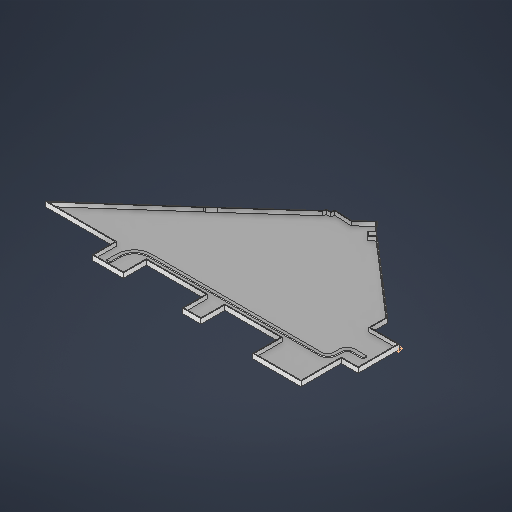
# Autodesk Inventor part: CIT-Floor-2
Saved by Autodesk Inventor 2026.1 (Build 301233020, 233B)
## iProperties
Created: 2025-10-17
Part Number: CIT-Floor-2
Material: Generic
Document SubType Name: Modeling
Designer: eduar
Density: 1 g/cm^3
Appearance: Default
Author: eduar
Autodesk Inventor part; units mm, degrees
ref_plane "YZ Plane" through (0, 0, 0) normal (1, 0, 0) x (0, 1, 0)
ref_plane "XZ Plane" through (0, 0, 0) normal (0, 1, 0) x (-1, 0, 0)
ref_plane "XY Plane" through (0, 0, 0) normal (0, 0, 1) x (1, 0, 0)
sketch "Sketch3" plane through (0, 0, 0) normal (0, 1, 0) x (-1, 0, 0)
  line L0 (0, 10031.5014) -> (4309.3277, 10031.5014)
  line L1 (4309.3277, 10031.5014) -> (4309.3277, 20253.6648)
  line L2 (16182.1297, 20253.6648) -> (4309.3277, 20253.6648)
  line L3 (16182.1297, 13144.1594) -> (16182.1297, 20253.6648)
  line L4 (0, 10031.5014) -> (0, 0)
  line L5 (0, 0) -> (7328.3017, 0)
  line L6 (7328.3017, -4479.3991) -> (7328.3017, 0)
  line L7 (7328.3017, -4479.3991) -> (26439.8438, -20982.2659)
  line L8 (26439.8438, -20982.2659) -> (27514.1147, -19948.948)
  line L9 (27514.1147, -19948.948) -> (28683.7243, -21071.6922)
  line L10 (27775.3508, -22022.2319) -> (28683.7243, -21071.6922)
  line L11 (27775.3508, -22022.2319) -> (29693.6379, -24167.9805)
  line L12 (29693.6379, -24167.9805) -> (32967.4576, -21145.3793)
  line L13 (32967.4576, -21145.3793) -> (37377.4906, -21381.4102)
  line L14 (37377.4906, -21381.4102) -> (37524.0883, -20493.0402)
  line L15 (38604.8798, -20527.5304) -> (37524.0883, -20493.0402)
  line L16 (38604.8798, -20527.5304) -> (38871.047, -19708.2796)
  line L17 (38871.047, -19708.2796) -> (39143.6329, -19289.1159)
  line L18 (39143.6329, -19289.1159) -> (52592.2756, -7382.5123)
  line L19 (38871.047, -19708.2796) -> (52965.6227, -7049.9272)
  line L20 (52965.6227, -7049.9272) -> (54462.7042, -5723.7531)
  line L21 (54850.5695, -5375.3135) -> (54462.7042, -5723.7531)
  line L22 (75709.6936, 13144.1594) -> (54850.5695, -5375.3135)
  line L23 (75709.6936, 13144.1594) -> (58320.151, 13144.1594)
  line L24 (58320.151, 13144.1594) -> (58320.151, 18979.1233)
  line L25 (50758.8526, 18979.1233) -> (58320.151, 18979.1233)
  line L26 (50758.8526, 13144.1594) -> (50758.8526, 18979.1233)
  line L27 (50758.8526, 13144.1594) -> (35157.7821, 13144.1594)
  line L28 (35157.7821, 19212.683) -> (35157.7821, 13144.1594)
  line L29 (30800.956, 19212.683) -> (35157.7821, 19212.683)
  line L30 (30800.956, 13144.1594) -> (30800.956, 19212.683)
  line L31 (30800.956, 13144.1594) -> (16182.1297, 13144.1594)
  dimension "d0" = 10031.5014
  dimension "d1" = 4309.3277
  dimension "d2" = 7328.3017
  dimension "d3" = 10222.1634
  dimension "d4" = 11872.802
  dimension "d5" = 7109.5054
  dimension "d6" = 14618.8263
  dimension "d7" = 15601.0705
  dimension "d8" = 6068.5236
  dimension "d9" = 6068.5236
  dimension "d10" = 4356.826
  dimension "d11" = 5834.964
  dimension "d12" = 7561.2984
  dimension "d13" = 17389.5426
  constraints: 64 end point, 15 perpendicular, 2 collinear
  measures "d0" distance of L0.start L4.end
  measures "d1" distance of L0.start L0.end
  measures "d2" distance of L4.end L5.end
  measures "d3" distance of L0.end L1.end
  measures "d4" distance of L2.start L1.end
  measures "d5" distance of L3.start L2.start
  measures "d6" distance of L30.start L3.start
  measures "d7" distance of L26.start L27.end
  measures "d8" distance of L30.start L29.start
  measures "d9" distance of L28.start L27.end
  measures "d10" distance of L29.start L28.start
  measures "d11" distance of L26.start L25.start
  measures "d12" distance of L25.start L24.end
  measures "d13" distance of L22.start L23.end
extrude "Extrusion1" add sketch "Sketch3" along normal blind 1000
shell "Shell1" thickness 200 outward yes removed faces 1 at (-21881.1241, 1000, -3761.3959)
sketch "Sketch4" plane through (-75709.6936, 0, 13144.1594) normal (0, 1, 0) x (1, 0, 0)
  line L0 (73643.0799, 7322.0862) -> (70709.8218, 7322.0862)
  arc A0 (70709.8218, 7322.0862) -> (68665.4298, 5277.2004) centre (70709.8218, 5277.6942) ccw
  line L1 (68665.4298, 5277.2004) -> (68665.4298, 3766.6003)
  arc A1 (67287.7087, 2388.8792) -> (68665.4298, 3766.6003) centre (67287.7087, 3766.6003) ccw
  line L2 (67287.7087, 2388.8792) -> (23771.1738, 2388.8792)
  arc A2 (23771.1738, 2388.8792) -> (19436.6359, -1949.6842) centre (23771.1738, -1945.6605) ccw
  line L3 (19436.6359, -1949.6842) -> (19436.6359, -4577.8792)
  line L4 (19436.6359, -4577.8792) -> (20327.3881, -4577.8792)
  line L5 (20327.3881, -4577.8792) -> (20327.3881, -1949.6842)
  arc A3 (23677.5205, 1655.3274) -> (20327.3881, -1949.6842) centre (23942.0953, -1949.6842) ccw
  line L6 (23677.5205, 1655.3274) -> (67287.7087, 1655.3274)
  arc A4 (67287.7087, 1655.3274) -> (69531.9829, 3907.8226) centre (67287.7087, 3899.6166) ccw
  line L7 (69531.9979, 3899.6166) -> (69531.9979, 5277.2004)
  arc A5 (70607.9309, 6428.1667) -> (69531.9979, 5277.2004) centre (70685.5804, 5277.2004) ccw
  line L8 (70516.5965, 6418.339) -> (73643.0799, 6418.339)
  line L9 (73643.0799, 6418.339) -> (73643.0799, 7322.0862)
  point P0 (75709.6936, 13144.1594)
  constraints: 20 end point, 14 point on circle, 7 tangent, 6 centre point, 3 horizontal, 3 perpendicular, 3 vertical, 1 parallel
extrude "Extrusion2" add sketch "Sketch4" along normal blind 300
body "Solid1"
